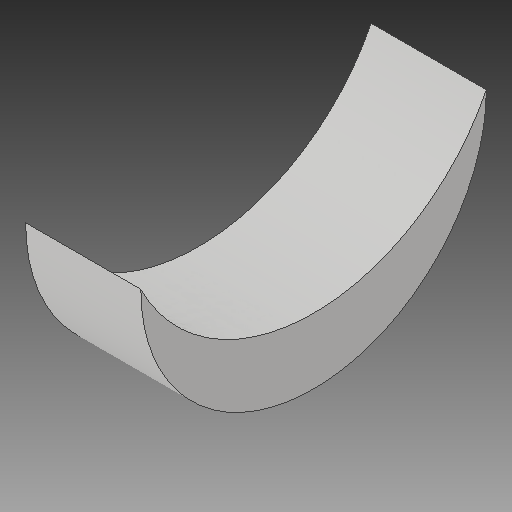
# Autodesk Inventor part: Tapa
Saved by Autodesk Inventor 2019 (Build 230136000, 136)
## iProperties
Created: 2020-01-21
Part Number: Tapa
Material: Generic
Document SubType Name: Modeling
Designer: peter
Density: 1 g/cm^3
Appearance: Default
Author: peter
Autodesk Inventor part; units mm, degrees
ref_plane "YZ Plane" through (0, 0, 0) normal (1, 0, 0) x (0, 1, 0)
ref_plane "XZ Plane" through (0, 0, 0) normal (0, 1, 0) x (-1, 0, 0)
ref_plane "XY Plane" through (0, 0, 0) normal (0, 0, 1) x (1, 0, 0)
sketch "Sketch2" plane through (0, 0, 0) normal (1, 0, 0) x (0, 1, 0)
  arc A0 (7.679, -6.681) -> (7.679, -15.681) centre (9.9085, -11.181) ccw
  arc A1 (7.679, -6.681) -> (7.679, -15.681) centre (7.679, -11.181) ccw
  point P0 (0, 0)
  dimension "d6" = 4.5
  constraints: 4 point on circle, 2 centre point
  measures "d6" radius of A1
extrude "Extrusion2" add sketch "Sketch2" along normal blind 3
body "Solid2"
